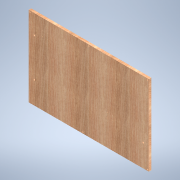
# Autodesk Inventor part: Seite
Saved by Autodesk Inventor 2021 (Build 250183000, 183)
## iProperties
Created: 2022-06-26
Part Number: Seite
Material: Holz (Birke)
Document SubType Name: Modeling
Designer: adria
Density: 0.55 g/cm^3
Appearance: Birke - natur - poliert
Mass: 3295.22 g
Surface Area: 7936.38 cm^2
Volume: 5991.3 cm^3
Author: adria
Autodesk Inventor part; units mm, degrees
ref_plane "YZ Plane" through (0, 0, 0) normal (1, 0, 0) x (0, 1, 0)
ref_plane "XZ Plane" through (0, 0, 0) normal (0, 1, 0) x (-1, 0, 0)
ref_plane "XY Plane" through (0, 0, 0) normal (0, 0, 1) x (1, 0, 0)
sketch "Skizze1" plane through (0, 0, 0) normal (0, 0, 1) x (1, 0, 0)
  line L0 (-375, -250) -> (375, -250)
  line L1 (375, -250) -> (375, 250)
  line L2 (375, 250) -> (-375, 250)
  line L3 (-375, 250) -> (-375, -250)
  line L4 (-375, -250) -> (375, 250) construction
  line L5 (375, -250) -> (-375, 250) construction
  point P0 (0, 0)
  dimension "d0" = 750
  dimension "d1" = 500
  constraints: 12 end point, 2 midpoint, 2 parallel, 1 horizontal, 1 perpendicular
  measures "d0" distance of L2.end L1.end
  measures "d1" distance of L1.end L0.end
extrude "Extrusion1" add sketch "Skizze1" along normal blind 16
sketch "Skizze5" plane through (0, 0, 16) normal (0, 0, 1) x (1, 0, 0)
  line L0 (375, -250) -> (375, 250) projected
  line L1 (375, 250) -> (-375, 250) projected
  line L2 (-375, 250) -> (-375, -250) projected
  line L3 (-375, -250) -> (375, -250) projected
  point P0 (0, 0)
  point P1 (340, -110)
  point P2 (-340, -110)
  point P3 (-340, 130)
  dimension "d39" = 140
  dimension "d40" = 140
  dimension "d41" = 35
  dimension "d42" = 35
  dimension "d44" = 120
  dimension "d57" = 35
  measures "d39" distance from line of L3 point (-340, -110)
  measures "d40" distance from line of L3 point (340, -110)
  measures "d41" distance from line of L0 point (340, -110)
  measures "d42" distance from line of L2 point (-340, -110)
  measures "d44" distance from line of L1 point (-340, 130)
  measures "d57" distance from line of L2 point (-340, 130)
hole "Bohrung4" at (340, -110, 16) at (-340, -110, 16) at (-340, 130, 16) direction (0, 0, -1) diameter 10 end through all
sketch "Skizze6" plane through (0, 0, 16) normal (0, 0, 1) x (1, 0, 0)
  circle A0 centre (-340, 130) radius 5 projected
  point P0 (0, 0)
  point P1 (-290, 149)
  point P2 (-259, 149)
  point P3 (-259, 180)
  point P4 (-290, 180)
  dimension "d59" = 31
  dimension "d60" = 31
  dimension "d65" = 50
  dimension "d66" = 50
  constraints: 2 horizontal alignment, 2 vertical alignment
  measures "d59" distance of point (-259, 149) point (-290, 149)
  measures "d60" distance of point (-259, 149) point (-259, 180)
  measures "d65" horizontal distance of A0.centre point (-290, 180)
  measures "d66" horizontal distance of A0.centre point (-290, 180)
hole "Bohrung5" at (-290, 149, 16) at (-259, 149, 16) at (-259, 180, 16) at (-290, 180, 16) direction (0, 0, -1) diameter 3 end through all
sketch "Skizze8" plane through (0, 0, 16) normal (0, 0, 1) x (1, 0, 0)
  line L0 (375, -250) -> (375, 250) projected
  line L1 (-375, -250) -> (375, -250) projected
  point P0 (0, 0)
  point P1 (114.5, -59)
  point P2 (145.5, -59)
  point P3 (114.5, -90)
  point P4 (145.5, -90)
  dimension "d85" = 31
  dimension "d86" = 31
  dimension "d87" = 160
  dimension "d88" = 229.5
  constraints: 2 horizontal alignment, 2 vertical alignment
  measures "d85" distance of point (114.5, -59) point (114.5, -90)
  measures "d86" distance of point (114.5, -90) point (145.5, -90)
  measures "d87" distance from line of L1 point (114.5, -90)
  measures "d88" distance from line of L0 point (145.5, -59)
hole "Bohrung7" at (114.5, -59, 16) at (145.5, -59, 16) at (114.5, -90, 16) at (145.5, -90, 16) direction (0, 0, -1) diameter 3 end through all
sketch "Skizze9" plane through (0, 0, 16) normal (0, 0, 1) x (1, 0, 0)
  line L0 (375, -250) -> (375, 250) projected
  line L1 (375, 250) -> (-375, 250) projected
  line L2 (-375, 250) -> (-375, -250) projected
  line L3 (-375, -250) -> (375, -250) projected
  point P0 (0, 0)
  point P1 (-367, 242)
  point P2 (0, 242)
  point P3 (367, 242)
  point P4 (367, -242)
  point P5 (-37, -242)
  dimension "d96" = 8
  dimension "d97" = 8
  dimension "d98" = 8
  dimension "d99" = 8
  dimension "d107" = 338
  constraints: 3 horizontal alignment, 2 vertical alignment
  measures "d96" distance from line of L1 point (-367, 242)
  measures "d97" distance from line of L2 point (-367, 242)
  measures "d98" distance from line of L0 point (367, 242)
  measures "d99" distance from line of point (-37, -242) L3
  measures "d107" distance from line of L2 point (-37, -242)
hole "Bohrung8" at (-367, 242, 16) at (0, 242, 16) at (367, 242, 16) at (367, -242, 16) at (-37, -242, 16) direction (0, 0, -1) diameter 8 depth 20 tip angle 118
equation "\"d98\" = d97"
equation "\"d99\" = d96"
